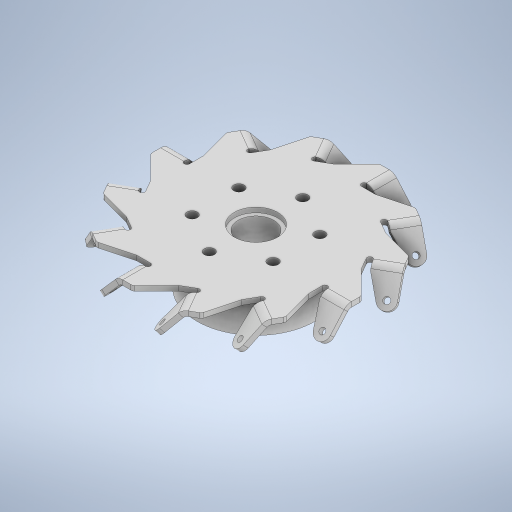
# Autodesk Inventor part: Part1
Saved by Autodesk Inventor 2024 (Build 280153000, 153)
## iProperties
Created: 2023-12-18
Part Number: Part1
Material: Generic
Document SubType Name: Sheet Metal
Designer: SAHITYA
Density: 1 g/cm^3
Sheet Metal Rule: Default
Appearance: Default
Author: SAHITYA
Autodesk Inventor part; units mm, degrees
ref_plane "YZ Plane" through (0, 0, 0) normal (1, 0, 0) x (0, 1, 0)
ref_plane "XZ Plane" through (0, 0, 0) normal (0, 1, 0) x (-1, 0, 0)
ref_plane "XY Plane" through (0, 0, 0) normal (0, 0, 1) x (1, 0, 0)
sketch "Sketch1" plane through (0, 0, 0) normal (0, 1, 0) x (-1, 0, 0)
  arc A0 (-25.657, -58.0859) -> (-51.2626, -37.4753) centre (0, 0) ccw
  circle A1 centre (0, 0) radius 9
  circle A2 centre (0, 0) radius 23.75 construction
  line L0 (-80.4985, 79.2379) -> (125.7878, 79.2379) construction
  line L1 (125.7878, 79.2379) -> (125.7878, -72.9015) construction
  line L2 (125.7878, -72.9015) -> (-80.4985, -72.9015) construction
  line L3 (-80.4985, -72.9015) -> (-80.4985, 79.2379) construction
  line L4 (43.6828, -16.9758) -> (43.6828, -9.9029)
  arc A3 (46.3191, -9.9029) -> (43.6828, -9.9029) centre (45.0009, -9.9029) ccw
  line L5 (46.0719, 7.3863) -> (57.5001, -4.0418)
  line L6 (58.0859, -18.9691) -> (58.0859, -5.456)
  arc A4 (58.0859, -5.456) -> (57.5001, -4.0418) centre (56.0859, -5.456) ccw
  line L7 (46.3191, -9.9029) -> (46.3191, -13.4394)
  line L8 (58.0859, -13.4394) -> (58.0859, -23.1894)
  line L9 (58.0859, -23.1894) -> (58.0859, -25.657)
  line L10 (50.1233, -23.1894) -> (49.8678, -23.1894)
  circle A5 centre (54.1046, -23.1894) radius 3.9813
  circle A6 centre (54.1046, -23.1894) radius 1.5
  line L11 (46.3191, -13.4394) -> (50.3634, -24.551)
  line L12 (69.3165, 131.516) -> (145.3862, -0.2407) construction
  line L13 (-33.263, -103.3838) -> (-109.3327, 28.3728) construction
  line L14 (145.3862, -0.2407) -> (-33.263, -103.3838) construction
  line L15 (-109.3327, 28.3728) -> (69.3165, 131.516) construction
  line L16 (46.3183, 7.1399) -> (42.7819, 13.2653)
  line L17 (45.0649, 14.5834) -> (46.8332, 11.5207)
  arc A7 (45.0649, 14.5834) -> (42.7819, 13.2653) centre (43.9234, 13.9243) ccw
  line L18 (36.2063, 29.4327) -> (51.8174, 25.2497)
  line L19 (57.0235, 17.4041) -> (61.8985, 8.9604)
  line L20 (59.7884, 12.6152) -> (53.0318, 24.3179)
  arc A8 (53.0318, 24.3179) -> (51.8174, 25.2497) centre (51.2998, 23.3179) ccw
  line L21 (55.0027, 4.9791) -> (54.7815, 4.8513)
  line L22 (46.8332, 11.5207) -> (55.8915, 3.9199)
  circle A9 centre (58.4506, 6.9697) radius 1.5
  circle A10 centre (58.4506, 6.9697) radius 3.9813
  line L23 (61.8985, 8.9604) -> (63.1323, 6.8233)
  line L24 (-5.7282, 148.5544) -> (126.0285, 72.4847) construction
  line L25 (22.8853, -106.1645) -> (-108.8713, -30.0948) construction
  line L26 (126.0285, 72.4847) -> (22.8853, -106.1645) construction
  line L27 (-108.8713, -30.0948) -> (-5.7282, 148.5544) construction
  line L28 (36.5429, 29.3425) -> (30.4176, 32.879)
  line L29 (31.7357, 35.1621) -> (34.7984, 33.3938)
  arc A11 (31.7357, 35.1621) -> (30.4176, 32.879) centre (31.0766, 34.0205) ccw
  line L30 (16.6392, 43.5926) -> (32.2503, 47.7756)
  line L31 (40.6817, 43.5841) -> (49.1255, 38.7091)
  line L32 (45.4706, 40.8193) -> (33.768, 47.5758)
  arc A12 (33.768, 47.5758) -> (32.2503, 47.7756) centre (32.768, 45.8438) ccw
  line L33 (45.1442, 31.8134) -> (45.0165, 31.5921)
  line L34 (34.7984, 33.3938) -> (46.4435, 31.3405)
  circle A13 centre (47.1349, 35.2613) radius 1.5
  circle A14 centre (47.1349, 35.2613) radius 3.9813
  line L35 (49.1255, 38.7091) -> (51.2626, 37.4753)
  line L36 (-79.2379, 125.7878) -> (72.9015, 125.7878) construction
  line L37 (72.9015, -80.4985) -> (-79.2379, -80.4985) construction
  line L38 (72.9015, 125.7878) -> (72.9015, -80.4985) construction
  line L39 (-79.2379, -80.4985) -> (-79.2379, 125.7878) construction
  line L40 (16.9758, 43.6828) -> (9.9029, 43.6828)
  line L41 (9.9029, 46.3191) -> (13.4394, 46.3191)
  arc A15 (9.9029, 46.3191) -> (9.9029, 43.6828) centre (9.9029, 45.0009) ccw
  line L42 (-7.3863, 46.0719) -> (4.0418, 57.5001)
  line L43 (13.4394, 58.0859) -> (23.1894, 58.0859)
  line L44 (18.9691, 58.0859) -> (5.456, 58.0859)
  arc A16 (5.456, 58.0859) -> (4.0418, 57.5001) centre (5.456, 56.0859) ccw
  line L45 (23.1894, 50.1233) -> (23.1894, 49.8678)
  line L46 (13.4394, 46.3191) -> (24.551, 50.3634)
  circle A17 centre (23.1894, 54.1046) radius 1.5
  circle A18 centre (23.1894, 54.1046) radius 3.9813
  line L47 (23.1894, 58.0859) -> (25.657, 58.0859)
  line L48 (-131.516, 69.3165) -> (0.2407, 145.3862) construction
  line L49 (103.3838, -33.263) -> (-28.3728, -109.3327) construction
  line L50 (0.2407, 145.3862) -> (103.3838, -33.263) construction
  line L51 (-28.3728, -109.3327) -> (-131.516, 69.3165) construction
  line L52 (-7.1399, 46.3183) -> (-13.2653, 42.7819)
  line L53 (-14.5834, 45.0649) -> (-11.5207, 46.8332)
  arc A19 (-14.5834, 45.0649) -> (-13.2653, 42.7819) centre (-13.9243, 43.9234) ccw
  line L54 (-29.4327, 36.2063) -> (-25.2497, 51.8174)
  line L55 (-17.4041, 57.0235) -> (-8.9604, 61.8985)
  line L56 (-12.6152, 59.7884) -> (-24.3179, 53.0318)
  arc A20 (-24.3179, 53.0318) -> (-25.2497, 51.8174) centre (-23.3179, 51.2998) ccw
  line L57 (-4.9791, 55.0027) -> (-4.8513, 54.7815)
  line L58 (-11.5207, 46.8332) -> (-3.9199, 55.8915)
  circle A21 centre (-6.9697, 58.4506) radius 1.5
  circle A22 centre (-6.9697, 58.4506) radius 3.9813
  line L59 (-8.9604, 61.8985) -> (-6.8233, 63.1323)
  line L60 (-148.5544, -5.7282) -> (-72.4847, 126.0285) construction
  line L61 (106.1645, 22.8853) -> (30.0948, -108.8713) construction
  line L62 (-72.4847, 126.0285) -> (106.1645, 22.8853) construction
  line L63 (30.0948, -108.8713) -> (-148.5544, -5.7282) construction
  line L64 (-29.3425, 36.5429) -> (-32.879, 30.4176)
  line L65 (-35.1621, 31.7357) -> (-33.3938, 34.7984)
  arc A23 (-35.1621, 31.7357) -> (-32.879, 30.4176) centre (-34.0205, 31.0766) ccw
  line L66 (-43.5926, 16.6392) -> (-47.7756, 32.2503)
  line L67 (-43.5841, 40.6817) -> (-38.7091, 49.1255)
  line L68 (-40.8193, 45.4706) -> (-47.5758, 33.768)
  arc A24 (-47.5758, 33.768) -> (-47.7756, 32.2503) centre (-45.8438, 32.768) ccw
  line L69 (-31.8134, 45.1442) -> (-31.5921, 45.0165)
  line L70 (-33.3938, 34.7984) -> (-31.3405, 46.4435)
  circle A25 centre (-35.2613, 47.1349) radius 1.5
  circle A26 centre (-35.2613, 47.1349) radius 3.9813
  line L71 (-38.7091, 49.1255) -> (-37.4753, 51.2626)
  line L72 (-125.7878, -79.2379) -> (-125.7878, 72.9015) construction
  line L73 (80.4985, 72.9015) -> (80.4985, -79.2379) construction
  line L74 (-125.7878, 72.9015) -> (80.4985, 72.9015) construction
  line L75 (80.4985, -79.2379) -> (-125.7878, -79.2379) construction
  line L76 (-43.6828, 16.9758) -> (-43.6828, 9.9029)
  line L77 (-46.3191, 9.9029) -> (-46.3191, 13.4394)
  arc A27 (-46.3191, 9.9029) -> (-43.6828, 9.9029) centre (-45.0009, 9.9029) ccw
  line L78 (-46.0719, -7.3863) -> (-57.5001, 4.0418)
  line L79 (-58.0859, 13.4394) -> (-58.0859, 23.1894)
  line L80 (-58.0859, 18.9691) -> (-58.0859, 5.456)
  arc A28 (-58.0859, 5.456) -> (-57.5001, 4.0418) centre (-56.0859, 5.456) ccw
  line L81 (-50.1233, 23.1894) -> (-49.8678, 23.1894)
  line L82 (-46.3191, 13.4394) -> (-50.3634, 24.551)
  circle A29 centre (-54.1046, 23.1894) radius 1.5
  circle A30 centre (-54.1046, 23.1894) radius 3.9813
  line L83 (-58.0859, 23.1894) -> (-58.0859, 25.657)
  line L84 (-69.3165, -131.516) -> (-145.3862, 0.2407) construction
  line L85 (33.263, 103.3838) -> (109.3327, -28.3728) construction
  line L86 (-145.3862, 0.2407) -> (33.263, 103.3838) construction
  line L87 (109.3327, -28.3728) -> (-69.3165, -131.516) construction
  line L88 (-46.3183, -7.1399) -> (-42.7819, -13.2653)
  line L89 (-45.0649, -14.5834) -> (-46.8332, -11.5207)
  arc A31 (-45.0649, -14.5834) -> (-42.7819, -13.2653) centre (-43.9234, -13.9243) ccw
  line L90 (-36.2063, -29.4327) -> (-51.8174, -25.2497)
  line L91 (-57.0235, -17.4041) -> (-61.8985, -8.9604)
  line L92 (-59.7884, -12.6152) -> (-53.0318, -24.3179)
  arc A32 (-53.0318, -24.3179) -> (-51.8174, -25.2497) centre (-51.2998, -23.3179) ccw
  line L93 (-55.0027, -4.9791) -> (-54.7815, -4.8513)
  line L94 (-46.8332, -11.5207) -> (-55.8915, -3.9199)
  circle A33 centre (-58.4506, -6.9697) radius 1.5
  circle A34 centre (-58.4506, -6.9697) radius 3.9813
  line L95 (-61.8985, -8.9604) -> (-63.1323, -6.8233)
  line L96 (5.7282, -148.5544) -> (-126.0285, -72.4847) construction
  line L97 (-22.8853, 106.1645) -> (108.8713, 30.0948) construction
  line L98 (-126.0285, -72.4847) -> (-22.8853, 106.1645) construction
  line L99 (108.8713, 30.0948) -> (5.7282, -148.5544) construction
  line L100 (-36.5429, -29.3425) -> (-30.4176, -32.879)
  line L101 (-31.7357, -35.1621) -> (-34.7984, -33.3938)
  arc A35 (-31.7357, -35.1621) -> (-30.4176, -32.879) centre (-31.0766, -34.0205) ccw
  line L102 (-16.6392, -43.5926) -> (-32.2503, -47.7756)
  line L103 (-40.6817, -43.5841) -> (-49.1255, -38.7091)
  line L104 (-45.4706, -40.8193) -> (-33.768, -47.5758)
  arc A36 (-33.768, -47.5758) -> (-32.2503, -47.7756) centre (-32.768, -45.8438) ccw
  line L105 (-45.1442, -31.8134) -> (-45.0165, -31.5921)
  line L106 (-34.7984, -33.3938) -> (-46.4435, -31.3405)
  circle A37 centre (-47.1349, -35.2613) radius 1.5
  circle A38 centre (-47.1349, -35.2613) radius 3.9813
  line L107 (-49.1255, -38.7091) -> (-51.2626, -37.4753)
  line L108 (79.2379, -125.7878) -> (-72.9015, -125.7878) construction
  line L109 (-72.9015, 80.4985) -> (79.2379, 80.4985) construction
  line L110 (-72.9015, -125.7878) -> (-72.9015, 80.4985) construction
  line L111 (79.2379, 80.4985) -> (79.2379, -125.7878) construction
  line L112 (-16.9758, -43.6828) -> (-9.9029, -43.6828)
  line L113 (-9.9029, -46.3191) -> (-13.4394, -46.3191)
  arc A39 (-9.9029, -46.3191) -> (-9.9029, -43.6828) centre (-9.9029, -45.0009) ccw
  line L114 (7.3863, -46.0719) -> (-4.0418, -57.5001)
  line L115 (-13.4394, -58.0859) -> (-23.1894, -58.0859)
  line L116 (-18.9691, -58.0859) -> (-5.456, -58.0859)
  arc A40 (-5.456, -58.0859) -> (-4.0418, -57.5001) centre (-5.456, -56.0859) ccw
  line L117 (-23.1894, -50.1233) -> (-23.1894, -49.8678)
  line L118 (-13.4394, -46.3191) -> (-24.551, -50.3634)
  circle A41 centre (-23.1894, -54.1046) radius 1.5
  circle A42 centre (-23.1894, -54.1046) radius 3.9813
  line L119 (-23.1894, -58.0859) -> (-25.657, -58.0859)
  line L120 (131.516, -69.3165) -> (-0.2407, -145.3862) construction
  line L121 (-103.3838, 33.263) -> (28.3728, 109.3327) construction
  line L122 (-0.2407, -145.3862) -> (-103.3838, 33.263) construction
  line L123 (28.3728, 109.3327) -> (131.516, -69.3165) construction
  line L124 (7.1399, -46.3183) -> (13.2653, -42.7819)
  line L125 (14.5834, -45.0649) -> (11.5207, -46.8332)
  arc A43 (14.5834, -45.0649) -> (13.2653, -42.7819) centre (13.9243, -43.9234) ccw
  line L126 (29.4327, -36.2063) -> (25.2497, -51.8174)
  line L127 (17.4041, -57.0235) -> (8.9604, -61.8985)
  line L128 (12.6152, -59.7884) -> (24.3179, -53.0318)
  arc A44 (24.3179, -53.0318) -> (25.2497, -51.8174) centre (23.3179, -51.2998) ccw
  line L129 (4.9791, -55.0027) -> (4.8513, -54.7815)
  line L130 (11.5207, -46.8332) -> (3.9199, -55.8915)
  circle A45 centre (6.9697, -58.4506) radius 1.5
  circle A46 centre (6.9697, -58.4506) radius 3.9813
  line L131 (8.9604, -61.8985) -> (6.8233, -63.1323)
  line L132 (148.5544, 5.7282) -> (72.4847, -126.0285) construction
  line L133 (-106.1645, -22.8853) -> (-30.0948, 108.8713) construction
  line L134 (72.4847, -126.0285) -> (-106.1645, -22.8853) construction
  line L135 (-30.0948, 108.8713) -> (148.5544, 5.7282) construction
  line L136 (29.3425, -36.5429) -> (32.879, -30.4176)
  line L137 (35.1621, -31.7357) -> (33.3938, -34.7984)
  arc A47 (35.1621, -31.7357) -> (32.879, -30.4176) centre (34.0205, -31.0766) ccw
  line L138 (43.5926, -16.6392) -> (47.7756, -32.2503)
  line L139 (43.5841, -40.6817) -> (38.7091, -49.1255)
  line L140 (40.8193, -45.4706) -> (47.5758, -33.768)
  arc A48 (47.5758, -33.768) -> (47.7756, -32.2503) centre (45.8438, -32.768) ccw
  line L141 (31.8134, -45.1442) -> (31.5921, -45.0165)
  line L142 (33.3938, -34.7984) -> (31.3405, -46.4435)
  circle A49 centre (35.2613, -47.1349) radius 1.5
  circle A50 centre (35.2613, -47.1349) radius 3.9813
  line L143 (38.7091, -49.1255) -> (37.4753, -51.2626)
  dimension "d0" = 127
  dimension "d1" = 18
  dimension "d2" = 47.5
  dimension "d42" = 135
  dimension "d43" = 2
  dimension "d46" = 9.75
  dimension "d48" = 45.001
  dimension "d49" = 3
  dimension "d53" = 360
  constraints: 192 end point, 75 point on circle, 51 centre point, 49 point on line, 15 coincident, 5 tangent, 5 vertical, 2 horizontal, 470 other
  measures "d0" diameter of A0
  measures "d1" diameter of A1
  measures "d2" diameter of A2
  measures "d42" angle of L6 L5
  measures "d43" radius of A4
  measures "d46" distance of L8.start L8.end
  measures "d48" horizontal distance of point (0, 0) A3.centre
  measures "d49" diameter of A6
extrude "Extrusion1" add sketch "Sketch1" along normal blind 2.5 contours A42 L117 L118 L113 A39 L112 L102 A36 L104 L103 A38 L105 L106 L101 A35 L100 L90 A32 L92 L91 A34 L93 L94 L89 A31 L88 L78 A28 L80 L79 A30 L81 L82 L77 A27 L76 L66 A24 L68 L67 A26 L69 L70 L65 A23 L64 L54 A20 L56 L55 A22 L57 L58 L53 A19 L52 L42 A16 L44 L43 A18 L45 L46 L41 A15 L40 L30 A12 L32 L31 A14 L33 L34 L29 A11 L28 L18 A8 L20 L19 A10 L21 L22 L17 A7 L16 L5 A4 L6 L8 A5 L10 L11 L7 A3 L4 L138 A48 L140 L139 A50 L141 L142 L137 A47 L136 L126 A44 L128 L127 A46 L129 L130 L125 A43 L124 L114 A40 L116 L115 | A42 | A46 | L118 L117 A42 | A50 | L130 L129 A46 | A5 | L142 L141 A50 | A10 | A5 L11 L10 | A14 | A10 L22 L21 | A18 | A14 L34 L33 | A22 | A18 L46 L45 | A26 | A22 L58 L57 | A30 | A26 L70 L69 | A34 | L82 L81 A30 | A38 | L94 L93 A34 | L106 L105 A38
sketch "Sketch2" plane through (0, 2.5, 0) normal (0, 1, 0) x (1, 0, 0)
  arc A0 (46.3191, -9.9029) -> (43.6828, -9.9029) centre (45.0009, -9.9029) ccw projected
  line L0 (46.3191, -9.9029) -> (46.3191, -11.1529)
  line L1 (46.3191, -9.9029) -> (46.3191, -13.4394) projected
  line L2 (46.3191, -11.1529) -> (58.0859, -11.1529)
  line L3 (58.0859, -23.1894) -> (58.0859, -5.456) projected
  line L4 (45.6899, 13.5009) -> (55.8803, 19.3842)
  line L5 (32.8182, 34.5371) -> (38.7016, 44.7274)
  line L6 (11.1529, 46.3191) -> (11.1529, 58.0859)
  line L7 (-13.5009, 45.6899) -> (-19.3842, 55.8803)
  line L8 (-34.5371, 32.8182) -> (-44.7274, 38.7016)
  line L9 (-46.3191, 11.1529) -> (-58.0859, 11.1529)
  line L10 (-45.6899, -13.5009) -> (-55.8803, -19.3842)
  line L11 (-32.8182, -34.5371) -> (-38.7016, -44.7274)
  line L12 (-11.1529, -46.3191) -> (-11.1529, -58.0859)
  line L13 (13.5009, -45.6899) -> (19.3842, -55.8803)
  line L14 (34.5371, -32.8182) -> (44.7274, -38.7016)
  point P0 (0, 0)
  dimension "d61" = 1.25
  dimension "d64" = 360
  constraints: 26 end point, 2 point on line, 1 perpendicular, 37 other
  measures "d61" distance of L0.start L0.end
sketch "Sketch3" plane through (0, 0, 0) normal (0, -1, 0) x (1, 0, 0)
  arc A0 (43.6828, 9.9029) -> (46.3191, 9.9029) centre (45.0009, 9.9029) ccw projected
  line L0 (46.3191, 9.9029) -> (46.3191, 11.1529)
  line L1 (46.3191, 11.1529) -> (58.0859, 11.1529)
  line L2 (58.0859, 23.1894) -> (58.0859, 5.456) projected
  point P0 (0, 0)
  dimension "d66" = 1.25
  constraints: 4 end point, 1 perpendicular, 1 point on line, 1 tangent, 1 vertical
  measures "d66" distance of L0.start L0.end
fold "Fold1" angle 48.556 bend radius 2.5 thickness 2.5 k factor 0.44 line from (46.3191, 0, 11.1529) to (58.0859, 0, 11.1529) line at bend centre moving side (0, 0, 1) folds toward (0, -1, 0)
sketch "Sketch9" plane through (0, 0, 0) normal (0, -1, 0) x (1, 0, 0)
  point P0 (0, 0)
pattern_circular "Circular Pattern1" count 12 over 360 about axis through (0, -10, 0) along (0, 1, 0) of "Fold1"
sketch "Sketch10" plane through (0, 0, 0) normal (0, -1, 0) x (1, 0, 0)
  circle A0 centre (0, 0) radius 23.75
  circle A1 centre (0, -23.75) radius 2.6
  circle A2 centre (20.5681, -11.875) radius 2.6
  circle A3 centre (20.5681, 11.875) radius 2.6
  circle A4 centre (0, 23.75) radius 2.6
  circle A5 centre (-20.5681, 11.875) radius 2.6
  circle A6 centre (-20.5681, -11.875) radius 2.6
  circle A7 centre (0, 0) radius 11
  dimension "d112" = 47.5
  dimension "d113" = 5.2
  dimension "d116" = 360
  dimension "d118" = 22
  constraints: 7 centre point, 2 coincident, 1 vertical alignment, 15 other
  measures "d113" diameter of A1
  measures "d118" diameter of A7
extrude "Extrusion2" cut sketch "Sketch10" against normal through all contours A3 A0 | A0 A3 | A2 A0 | A0 A2 | A4 A0 | A0 A4 | A1 A0 | A0 A1 | A5 A0 | A0 A5 | A6 A0 | A0 A6
extrude "Extrusion3" cut sketch "Sketch10" against normal through all contours A7
sketch "Sketch11" plane through (0, 0, 0) normal (0, -1, 0) x (1, 0, 0)
  circle A0 centre (0, 0) radius 9
  circle A1 centre (0, 0) radius 30
  circle A2 centre (20.5681, 11.875) radius 2.6 projected
  circle A3 centre (20.5681, 11.875) radius 2.6
  circle A4 centre (20.5681, -11.875) radius 2.6 projected
  circle A5 centre (20.5681, -11.875) radius 2.6
  circle A6 centre (0, -23.75) radius 2.6 projected
  circle A7 centre (0, -23.75) radius 2.6
  circle A8 centre (-20.5681, -11.875) radius 2.6 projected
  circle A9 centre (-20.5681, -11.875) radius 2.6
  circle A10 centre (-20.5681, 11.875) radius 2.6 projected
  circle A11 centre (-20.5681, 11.875) radius 2.6
  circle A12 centre (0, 23.75) radius 2.6 projected
  circle A13 centre (0, 23.75) radius 2.6
  dimension "d123" = 18
  dimension "d124" = 60
  constraints: 8 centre point, 8 coincident
  measures "d123" diameter of A0
  measures "d124" diameter of A1
extrude "Extrusion4" add sketch "Sketch11" along normal blind 25.023
body "Solid1"
